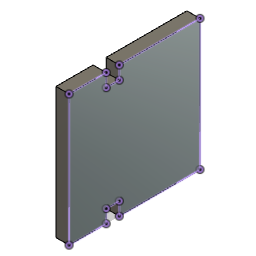
Sketch with parametric slot location v1 (Autodesk Fusion 360 design; units mm, degrees)
Autodesk Fusion 360 part; units mm, degrees
sketch "Sketch1" plane through (0, 0, 0) normal (1, 0, 0) x (0, 0, -1)
  line L0 (5, 37.5) -> (5, -12.5)
  line L1 (-45, -12.5) -> (-45, 37.5)
  line L2 (-25.8333, 37.5) -> (-25.8333, 32.5)
  line L3 (-25.8333, 32.5) -> (-30.8333, 32.5)
  line L4 (-30.8333, 32.5) -> (-30.8333, 37.5)
  line L5 (-25.8333, -12.5) -> (-25.8333, -7.5)
  line L6 (-25.8333, -7.5) -> (-30.8333, -7.5)
  line L7 (-30.8333, -7.5) -> (-30.8333, -12.5)
  line L8 (-45, 37.5) -> (-30.8333, 37.5)
  line L9 (-25.8333, 37.5) -> (5, 37.5)
  line L10 (5, -12.5) -> (-25.8333, -12.5)
  line L11 (-30.8333, -12.5) -> (-45, -12.5)
  dimension "d5" = 50
  dimension "d6" = 50
  dimension "d7" = 14.1667
  dimension "d8" = 5
  dimension "d9" = 5
  constraint horizontal L8
  constraint vertical L0
  constraint horizontal L10
  constraint vertical L1
  constraint vertical L2
  constraint horizontal L3
  constraint vertical L4
  constraint vertical L5
  constraint horizontal L6
  constraint vertical L7
  constraint coincident L7.end L10
  constraint collinear L8 L9
  constraint collinear L10 L11
  constraint equal L3 L6
  constraint collinear L4 L7
  constraint equal L4 L7
  measures "d5" distance of L0.end L1.start
  measures "d6" distance of L1.end L1.start
  measures "d7" distance of L1.end L4.end
  measures "d8" distance of L2.end L3.end
  measures "d9" distance of L4.end L3.end
extrude "Extrude1" add sketch "Sketch1" along normal blind 5
sketch "Sketch2" plane through (5, 0, 0) normal (1, 0, 0) x (0, 0, -1)
  line L0 (-25.8333, 37.5) -> (-25.8333, 32.5)
  line L1 (-25.8333, 32.5) -> (-30.8333, 32.5)
  line L2 (-30.8333, 32.5) -> (-30.8333, 37.5)
  line L3 (-30.8333, 37.5) -> (-45, 37.5)
  line L4 (-45, 37.5) -> (-45, -12.5)
  line L5 (-45, -12.5) -> (-30.8333, -12.5)
  line L6 (-30.8333, -12.5) -> (-30.8333, -7.5)
  line L7 (-30.8333, -7.5) -> (-25.8333, -7.5)
  line L8 (-25.8333, -7.5) -> (-25.8333, -12.5)
  line L9 (-25.8333, -12.5) -> (5, -12.5)
  line L10 (5, -12.5) -> (5, 37.5)
  line L11 (5, 37.5) -> (-25.8333, 37.5)
equation "w = 50 mm"
equation "h = 50 mm"
equation "sw = 5 mm"
equation "sd = 5 mm"
equation "d5 = w"
equation "d6 = h"
equation "d7 = ( 1 / 3 ) * w - ( 1 / 2 ) * sw"
equation "d8 = sw"
equation "d9 = sd"
